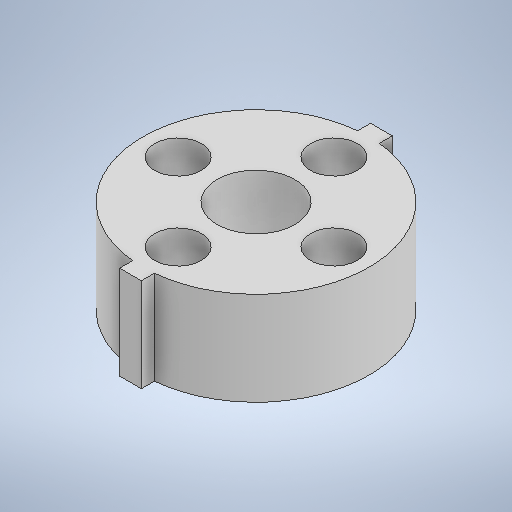
# Autodesk Inventor part: joy stick part 1
Saved by Autodesk Inventor 2025.2 (Build 292293000, 293)
## iProperties
Created: 2025-04-03
Part Number: joy stick part 1
Material: Generic
Document SubType Name: Modeling
Designer: avnr2
Density: 1 g/cm^3
Appearance: Default
Author: avnr2
Autodesk Inventor part; units mm, degrees
ref_plane "YZ Plane" through (0, 0, 0) normal (1, 0, 0) x (0, 1, 0)
ref_plane "XZ Plane" through (0, 0, 0) normal (0, 1, 0) x (-1, 0, 0)
ref_plane "XY Plane" through (0, 0, 0) normal (0, 0, 1) x (1, 0, 0)
sketch "Sketch1" plane through (0, 0, 0) normal (0, 1, 0) x (-1, 0, 0)
  circle A0 centre (0, 0) radius 7.25
  line L0 (0, -7.25) -> (0, -8.05)
  line L1 (0, -8.05) -> (0.7, -8.05)
  line L2 (0.7, -8.05) -> (0.7, -7.2161)
  line L3 (0, -8.05) -> (-0.7, -8.05)
  line L4 (-0.7, -8.05) -> (-0.7, -7.2161)
  line L5 (6.6169, 0) -> (-6.6879, 0)
  line L6 (0, 7.25) -> (0, 8.05)
  line L7 (0, 8.05) -> (0.7, 8.05)
  line L8 (0.7, 8.05) -> (0.7, 7.2161)
  line L9 (0, 8.05) -> (-0.7, 8.05)
  line L10 (-0.7, 8.05) -> (-0.7, 7.2161)
  point P0 (-0.7, 7.2161)
  dimension "d0" = 0.8
  dimension "d1" = 0.7
  dimension "d13" = 14.5
  constraints: 22 end point, 8 symmetric about line, 2 perpendicular, 2 point on circle, 1 centre point, 1 coincident, 1 horizontal, 1 vertical
  measures "d0" distance of L0.start L0.end
  measures "d1" distance of L0.end L1.end
  measures "d13" diameter of A0
extrude "Extrusion1" add sketch "Sketch1" along normal blind 6
sketch "Sketch2" plane through (0, 6, 0) normal (0, 1, 0) x (1, 0, 0)
  circle A0 centre (0, 0) radius 2.5
  circle A1 centre (0, 0) radius 5 construction
  circle A2 centre (-5, 0) radius 1.5
  circle A3 centre (0, 0) radius 5 construction
  circle A4 centre (0, -5) radius 1.5
  circle A5 centre (0, 0) radius 5 construction
  circle A6 centre (5, 0) radius 1.5
  circle A7 centre (0, 0) radius 5 construction
  circle A8 centre (0, 5) radius 1.5
  dimension "d5" = 10
  dimension "d4" = 5
  dimension "d6" = 3
  dimension "d9" = 360
  constraints: 5 centre point, 4 coincident, 2 horizontal alignment, 2 vertical alignment, 27 other
  measures "d4" diameter of A0
  measures "d6" diameter of A2
extrude "Extrusion2" cut sketch "Sketch2" against normal blind 6
body "Solid1"
